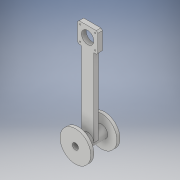
# Autodesk Inventor part: arm_proximal
Saved by Autodesk Inventor 2019 (Build 230136000, 136)
## iProperties
Created: 2019-05-16
Part Number: arm_proximal
Material: Generic
Document SubType Name: Modeling
Designer: Nathan
Density: 1 g/cm^3
Appearance: Default
Author: Nathan
Autodesk Inventor part; units mm, degrees
ref_plane "YZ Plane" through (0, 0, 0) normal (1, 0, 0) x (0, 1, 0)
ref_plane "XZ Plane" through (0, 0, 0) normal (0, 1, 0) x (-1, 0, 0)
ref_plane "XY Plane" through (0, 0, 0) normal (0, 0, 1) x (1, 0, 0)
sketch "Sketch1" plane through (0, 0, 0) normal (0, 0, 1) x (1, 0, 0)
  circle A0 centre (0, 0) radius 31.75
  dimension "shoulder_gear_diameter" = 63.5
  dimension "d0" = 63.5
  constraints: 2 coincident, 1 centre point
  measures "d0" diameter of A0
extrude "Extrusion1" add sketch "Sketch1" along normal blind 6.35
sketch "Sketch2" plane through (0, 0, 6.35) normal (0, 0, 1) x (1, 0, 0)
  circle A0 centre (0, 0) radius 12.7
  dimension "d14" = 25.4
  constraints: 1 centre point, 1 coincident
  measures "d14" diameter of A0
extrude "Extrusion2" add sketch "Sketch2" along normal blind 47.625
sketch "Sketch3" plane through (0, 0, 53.975) normal (0, 0, 1) x (1, 0, 0)
  circle A0 centre (0, 0) radius 31.75 projected
  circle A1 centre (0, 0) radius 31.75
  constraints: 1 centre point, 1 coincident, 1 concentric
extrude "Extrusion3" add sketch "Sketch3" along normal blind 6.35
hole "Hole1" at (0, 0, 0) direction (0, 0, 1) diameter 12.7 end through all
sketch "Sketch5" plane through (0, 0, 0) normal (0, 1, 0) x (-1, 0, 0)
  line L0 (6.35, 0) -> (6.35, 60.325) projected
  line L1 (12.7, 6.35) -> (12.7, 53.975) projected
  line L2 (-12.7, 6.35) -> (-12.7, 53.975) projected
  line L3 (12.7, 30.1625) -> (-12.7, 30.1625) construction
  line L4 (12.7, 34.925) -> (-12.7, 34.925)
  line L5 (-12.7, 34.925) -> (-12.7, 25.4)
  line L6 (-12.7, 25.4) -> (12.7, 25.4)
  line L7 (12.7, 25.4) -> (12.7, 34.925)
  point P0 (0, 0)
  dimension "d15" = 9.525
  constraints: 10 end point, 2 midpoint, 2 parallel, 2 point on line, 1 horizontal, 1 perpendicular, 1 other
  measures "d15" distance between parallel lines of L6 L4
extrude "Extrusion4" add sketch "Sketch5" along normal blind 161.2
sketch "Sketch6" plane through (0, 0, 34.925) normal (0, 0, 1) x (1, 0, 0)
  line L0 (-12.7, 161.2) -> (12.7, 161.2) projected
  line L1 (-21, 161.2) -> (21, 161.2)
  line L2 (21, 161.2) -> (21, 203.2)
  line L3 (21, 203.2) -> (-21, 203.2)
  line L4 (-21, 203.2) -> (-21, 161.2)
  line L5 (0, -78.74) -> (0, 250.19) projected
  point P0 (0, 0)
  dimension "d18" = 42
  constraints: 8 end point, 2 parallel, 2 perpendicular, 1 collinear, 1 horizontal, 1 other
  measures "d18" distance of L1.start L1.end
extrude "Extrusion5" add sketch "Sketch6" against normal blind 9.525
sketch "Sketch7" plane through (0, 0, 34.925) normal (0, 0, 1) x (1, 0, 0)
  line L0 (-21, 203.2) -> (-21, 161.2) projected
  line L1 (21, 203.2) -> (-21, 203.2) projected
  line L2 (21, 161.2) -> (21, 203.2) projected
  line L3 (-15.5, 166.7) -> (-15.5, 197.7)
  line L4 (-15.5, 197.7) -> (15.5, 197.7)
  line L5 (15.5, 197.7) -> (15.5, 166.7)
  circle A0 centre (0, 182.2) radius 12.7
  point P0 (0, 0)
  point P1 (15.5, 182.2)
  point P2 (0, 197.7)
  dimension "d21" = 5.5
  dimension "d22" = 31
  dimension "d23" = 25.4
  constraints: 6 end point, 4 coincident, 2 horizontal alignment, 2 midpoint, 1 centre point, 1 vertical alignment, 2 other
  measures "d21" distance between parallel lines of L1 L4
  measures "d22" distance of L3.start L3.end
  measures "d23" diameter of A0
extrude "Extrusion6" cut sketch "Sketch7" against normal blind 9.525
hole "Hole2" at (-15.5, 166.7, 34.925) at (15.5, 166.7, 34.925) at (15.5, 197.7, 34.925) at (-15.5, 197.7, 34.925) direction (0, 0, -1) diameter 2.5 end through all
chamfer "Chamfer1" distance 3.175 angle 45 4 edges at (-21, 203.2, 30.1625) (21, 203.2, 30.1625) (21, 161.2, 30.1625) (-21, 161.2, 30.1625)
equation "\"shoulder_gear_diameter\" = 63.5"
equation "\"d0\" = shoulder_gear_diameter"
equation "\"d1\" = shoulder_gear_thickness"
equation "\"d14\" = arm_proximal_central_diameter"
equation "\"d3\" = -2 * shoulder_wall_thickness + shoulder_width - 2 * shoulder_gear_thickness"
equation "\"d5\" = shoulder_gear_thickness"
equation "\"d7\" = shoulder_gear_shaft_diameter"
equation "\"d15\" = arm_proximal_thickness"
equation "\"d19\" = arm_proximal_thickness"
equation "\"d23\" = arm_proximal_motor_boss"
equation "\"d24\" = arm_proximal_thickness"
equation "\"base_length\" = 177.8"
equation "\"base_width\" = 127"
equation "\"base_height\" = 12.7"
equation "\"base_cutout_contact_angle\" = 70deg"
equation "\"base_cutout_diameter\" = 44.45"
equation "\"turntable_motor_support_thickness\" = 3.175"
equation "\"turntable_motor_support_width\" = 63.5"
equation "\"turntable_motor_support_height\" = 19.05"
equation "\"turntable_motor_boss\" = 25.4"
equation "\"turntable_bed_depth\" = 3.175"
equation "\"turntable_diameter\" = 101.6"
equation "\"turntable_height\" = 9.525"
equation "\"turntable_spur_width\" = 6.35"
equation "\"turntable_retention_shaft_diameter\" = 6.35"
equation "\"turntable_retention_shaft_length\" = 152.4"
equation "\"spine_diameter\" = 31.75"
equation "\"spine_height\" = 25.4"
equation "\"shoulder_length\" = 50.8"
equation "\"shoulder_width\" = 69.85"
equation "\"shoulder_wall_thickness\" = 4.7625"
equation "\"shoulder_gear_thickness\" = 6.35"
equation "\"shoulder_motor_gear_diameter\" = 25.4"
equation "\"shoulder_gear_shaft_diameter\" = 12.7"
equation "\"shoulder_motor_boss\" = 25.4"
equation "\"arm_proximal_length\" = 203.2"
equation "\"arm_proximal_central_diameter\" = 25.4"
equation "\"arm_distal_length\" = 152.4"
equation "\"arm_proximal_thickness\" = 9.525"
equation "\"arm_proximal_motor_boss\" = 25.4"
body "Solid1"
